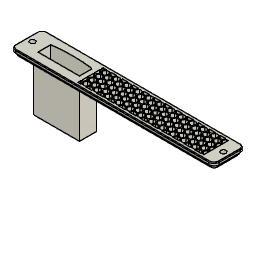
Front Vent -  SD_Card (Autodesk Fusion 360 design; units mm, degrees)
Autodesk Fusion 360 part; units mm, degrees
sketch "Sketch1" plane through (0, 0, 0) normal (0, 0, 1) x (1, 0, 0)
  line L0 (-84.9, 11.9) -> (84.9, 11.9)
  line L1 (84.9, 11.9) -> (84.9, -11.9)
  line L2 (84.9, -11.9) -> (-84.9, -11.9)
  line L3 (-84.9, -11.9) -> (-84.9, 11.9)
  circle A0 centre (-81.9, 8.9) radius 3
  circle A1 centre (-81.9, -8.9) radius 3
  circle A2 centre (81.9, 8.9) radius 3
  circle A3 centre (81.9, -8.9) radius 3
  line L4 (-107.1873, 0) -> (-105, 0)
  line L5 (-105, 0) -> (105, 0) construction
  circle A4 centre (-81, 0) radius 2.2
  circle A5 centre (81, 0) radius 2.2
  dimension "d21_3_1" = 169.8
  dimension "d22_3_1" = 84.9
  dimension "d23_3_1" = 23.8
  dimension "d24_3_1" = 11.9
  dimension "d25_3_1" = 6
  dimension "d26_3_1" = 6
  dimension "d27_3_1" = 6
  dimension "d28_3_1" = 6
  dimension "d29_3_1" = 210
  dimension "d30_3_1" = 4.4
  dimension "d31_3_1" = 4.4
  dimension "d32_3_1" = 3.9
  dimension "d33_3_1" = 3.9
  constraint horizontal L0
  constraint vertical L1
  constraint horizontal L2
  constraint vertical L3
  constraint tangent L0 A0
  constraint tangent L3 A0
  constraint tangent L2 A1
  constraint tangent L3 A1
  constraint tangent L2 A3
  constraint tangent L0 A2
  constraint tangent L1 A2
  constraint tangent L1 A3
  constraint parallel L2 L4
  constraint parallel L2 L5
  constraint midpoint origin L5
  constraint coincident L5 A4.centre
  constraint coincident L5 A5.centre
  measures "d21_3_1" distance of L0.start L0.end
  measures "d22_3_1" distance of origin L3
  measures "d23_3_1" distance of L0.start L2.end
  measures "d24_3_1" distance of origin L0
  measures "d25_3_1" diameter of A0
  measures "d26_3_1" diameter of A1
  measures "d27_3_1" diameter of A2
  measures "d28_3_1" diameter of A3
  measures "d29_3_1" distance of L4.end L5.end
  measures "d30_3_1" diameter of A4
  measures "d31_3_1" diameter of A5
  measures "d32_3_1" distance of L3 A4.centre
  measures "d33_3_1" distance of L1 A5.centre
extrude "Extrude1" add sketch "Sketch1" along normal blind 2.8 contours L0 L1 L2 L3 A0 A1 A2 A3 | A0 | A2 | A1 | A3
sketch "Sketch2" plane through (0, 0, 2.8) normal (0, 0, 1) x (-1, 0, 0)
  circle A0 centre (81, 0) radius 2.2
  circle A1 centre (-81, 0) radius 2.2
  arc A2 (81.9, -11.9) -> (84.9, -8.9) centre (81.9, -8.9) ccw
  line L0 (84.9, -8.9) -> (84.9, 8.9)
  arc A3 (84.9, 8.9) -> (81.9, 11.9) centre (81.9, 8.9) ccw
  line L1 (81.9, 11.9) -> (-81.9, 11.9)
  arc A4 (-81.9, 11.9) -> (-84.9, 8.9) centre (-81.9, 8.9) ccw
  line L2 (-84.9, 8.9) -> (-84.9, -8.9)
  arc A5 (-84.9, -8.9) -> (-81.9, -11.9) centre (-81.9, -8.9) ccw
  line L3 (-81.9, -11.9) -> (81.9, -11.9)
  line L4 (-81.9, -13.3) -> (81.9, -13.3)
  arc A6 (81.9, -13.3) -> (86.3, -8.9) centre (81.9, -8.9) ccw
  line L5 (86.3, -8.9) -> (86.3, 8.9)
  arc A7 (86.3, 8.9) -> (81.9, 13.3) centre (81.9, 8.9) ccw
  line L6 (81.9, 13.3) -> (-81.9, 13.3)
  arc A8 (-81.9, 13.3) -> (-86.3, 8.9) centre (-81.9, 8.9) ccw
  line L7 (-86.3, 8.9) -> (-86.3, -8.9)
  arc A9 (-86.3, -8.9) -> (-81.9, -13.3) centre (-81.9, -8.9) ccw
  dimension "d36_3_1" = 1.4
extrude "Extrude2" add sketch "Sketch2" along normal blind 2.4 contours A2 L0 A3 L1 A4 L2 A5 L3 | L4 A6 L5 A7 L6 A8 L7 A9
chamfer "Chamfer1" distance 0.6 angle 45 8 edges at (86.3, 0, 5.2) (85.0113, 12.0113, 5.2) (0, 13.3, 5.2) (-85.0113, 12.0113, 5.2) (-86.3, 0, 5.2) (-85.0113, -12.0113, 5.2) (0, -13.3, 5.2) (85.0113, -12.0113, 5.2)
sketch "Sketch4" plane through (-1.7827, -2.3697, 0) normal (0, 0, -1) x (1, 0, 0)
  circle A0 centre (-79.2173, -2.3697) radius 2.2
  circle A1 centre (82.7827, -2.3697) radius 2.2
  arc A2 (-83.1173, -11.2697) -> (-80.1173, -14.2697) centre (-80.1173, -11.2697) ccw
  line L0 (-80.1173, -14.2697) -> (83.6827, -14.2697)
  arc A3 (83.6827, -14.2697) -> (86.6827, -11.2697) centre (83.6827, -11.2697) ccw
  line L1 (86.6827, -11.2697) -> (86.6827, 6.5303)
  arc A4 (86.6827, 6.5303) -> (83.6827, 9.5303) centre (83.6827, 6.5303) ccw
  line L2 (83.6827, 9.5303) -> (-80.1173, 9.5303)
  arc A5 (-80.1173, 9.5303) -> (-83.1173, 6.5303) centre (-80.1173, 6.5303) ccw
  line L3 (-83.1173, 6.5303) -> (-83.1173, -11.2697)
  line L4 (-82.6173, 6.5303) -> (-82.6173, -11.2697)
  arc A6 (-82.6173, -11.2697) -> (-80.1173, -13.7697) centre (-80.1173, -11.2697) ccw
  line L5 (-80.1173, -13.7697) -> (83.6827, -13.7697)
  arc A7 (83.6827, -13.7697) -> (86.1827, -11.2697) centre (83.6827, -11.2697) ccw
  line L6 (86.1827, -11.2697) -> (86.1827, 6.5303)
  arc A8 (86.1827, 6.5303) -> (83.6827, 9.0303) centre (83.6827, 6.5303) ccw
  line L7 (83.6827, 9.0303) -> (-80.1173, 9.0303)
  arc A9 (-80.1173, 9.0303) -> (-82.6173, 6.5303) centre (-80.1173, 6.5303) ccw
  dimension "d44_3_1" = -0.5
extrude "Extrude4" cut sketch "Sketch4" against normal up to surface (2.8 mm away) contours A2 L0 A3 L1 A4 L2 A5 L3
sketch "Sketch6" plane through (0, 0, 5.2) normal (0, 0, 1) x (-1, 0, 0)
  circle A0 centre (81, 0) radius 2.2
  circle A1 centre (-81, 0) radius 2.2
  line L0 (-85.7, 8.9) -> (-85.7, -8.9)
  arc A2 (-85.7, -8.9) -> (-81.9, -12.7) centre (-81.9, -8.9) ccw
  line L1 (-81.9, -12.7) -> (81.9, -12.7)
  arc A3 (81.9, -12.7) -> (85.7, -8.9) centre (81.9, -8.9) ccw
  line L2 (85.7, -8.9) -> (85.7, 8.9)
  arc A4 (85.7, 8.9) -> (81.9, 12.7) centre (81.9, 8.9) ccw
  line L3 (81.9, 12.7) -> (-81.9, 12.7)
  arc A5 (-81.9, 12.7) -> (-85.7, 8.9) centre (-81.9, 8.9) ccw
  line L4 (71, -5.4) -> (35.8, -5.4)
  line L5 (35.8, -5.4) -> (35.8, 5.4)
  line L6 (35.8, 5.4) -> (71, 5.4)
  line L7 (71, 5.4) -> (71, -5.4)
  arc A6 (35.8, -5.4) -> (71, -5.4) centre (53.4, 123.0667) ccw
  arc A7 (33.8, -7.133) -> (73, -7.133) centre (53.4, 123.0667) ccw
  line L8 (73, 7.4) -> (73, -7.133)
  line L9 (33.8, 7.4) -> (73, 7.4)
  line L10 (33.8, -7.133) -> (33.8, 7.4)
  point P0 (81, 0)
  point P1 (71, 0)
  point P2 (53.4, 5.4)
  point P3 (53.4, -6.6)
  dimension "d323_1" = 12
  dimension "d324_1" = 10.8
  dimension "d325_1" = 10
  dimension "d326_1" = 2
  dimension "d337_1" = 35.2
  constraint horizontal L4
  constraint vertical L5
  constraint horizontal L6
  constraint vertical L7
  constraint coincident P0 A0.centre
  constraint midpoint L7 P1
  constraint midpoint L6 P2
  constraint midpoint A6 P3
  constraint horizontal P0 P1
  measures "d323_1" distance of P2 P3
  measures "d324_1" distance of L4.end L5.end
  measures "d325_1" distance of P0 P1
  measures "d337_1" distance of L5 L7
extrude "Extrude16" cut sketch "Sketch6" against normal blind 10 contours L4 A6
extrude "Extrude10" cut sketch "Sketch6" against normal blind 5.2 contours L4 L5 L6 L7
extrude "Extrude9" add sketch "Sketch6" against normal blind 44 contours A7 L8 L9 L10
sketch "Sketch7" plane through (0, 0, -38.8) normal (0, 0, -1) x (1, 0, 0)
  line L0 (-35.8, 5.4) -> (-35.8, -5.4)
  arc A0 (-71, -5.4) -> (-35.8, -5.4) centre (-53.4, 123.0667) ccw
  line L1 (-71, -5.4) -> (-71, 5.4)
  line L2 (-71, 5.4) -> (-35.8, 5.4)
  arc A1 (-73, -7.133) -> (-33.8, -7.133) centre (-53.4, 123.0667) ccw
  line L3 (-33.8, -7.133) -> (-33.8, 7.4)
  line L4 (-33.8, 7.4) -> (-73, 7.4)
  line L5 (-73, 7.4) -> (-73, -7.133)
extrude "Extrude11" add sketch "Sketch7" along normal blind 2 contours L0 A0 L1 L2 | A1 L3 L4 L5
sketch "Sketch8" plane through (0, 0, -40.8) normal (0, 0, -1) x (1, 0, 0)
  line L0 (-73, 7.4) -> (-73, -7.133)
  arc A0 (-73, -7.133) -> (-33.8, -7.133) centre (-53.4, 123.0667) ccw
  line L1 (-33.8, -7.133) -> (-33.8, 7.4)
  line L2 (-64.4, 2) -> (-42.4, 2)
  line L3 (-42.4, 2) -> (-42.4, -2)
  line L4 (-42.4, -2) -> (-64.4, -2)
  line L5 (-64.4, -2) -> (-64.4, 2)
  point P0 (-81, 0)
  point P1 (-64.4, 0)
  point P2 (-53.4, 2)
  point P3 (-53.4, 5.4)
  dimension "d335_1" = 13.8426
  dimension "d336_1" = 22
  dimension "d338_1" = 4
  constraint horizontal L2
  constraint vertical L3
  constraint horizontal L4
  constraint vertical L5
  constraint midpoint L5 P1
  constraint horizontal P0 P1
  constraint midpoint L2 P2
  constraint vertical P2 P3
  measures "d336_1" distance of L2.start L2.end
  measures "d338_1" distance of L2.end L3.end
extrude "Extrude12" cut sketch "Sketch8" against normal blind 2
fillet "Fillet1" radius 1 4 edges at (-64.4, -2, -39.8) (-42.4, -2, -39.8) (-42.4, 2, -39.8) (-64.4, 2, -39.8)
sketch "Sketch10" plane through (0, 0, 5.2) normal (0, 0, 1) x (-1, 0, 0)
  line L0 (31.8, -10.7) -> (-75, -10.7)
  line L1 (-75, -10.7) -> (-75, 10.7)
  line L2 (-75, 10.7) -> (31.8, 10.7)
  line L3 (31.8, 10.7) -> (31.8, -10.7)
  line L4 (33.8, -7.133) -> (33.8, 7.4)
  line L5 (-21.6, -10.7) -> (-21.6, 10.7) construction
  line L6 (81.9, 12.7) -> (-81.9, 12.7)
  line L7 (-81.9, -12.7) -> (81.9, -12.7)
  line L8 (29.1731, 0) -> (30.4865, -2.275)
  line L9 (30.4865, -2.275) -> (33.1135, -2.275)
  line L10 (33.1135, -2.275) -> (34.4269, 0)
  line L11 (34.4269, 0) -> (33.1135, 2.275)
  line L12 (33.1135, 2.275) -> (30.4865, 2.275)
  line L13 (30.4865, 2.275) -> (29.1731, 0)
  line L14 (31.8, 0) -> (29.0768, 0)
  line L15 (29.0768, 0) -> (-75, 0) construction
  line L16 (30.4865, -3.075) -> (29.1731, -5.35)
  line L17 (29.1731, -5.35) -> (30.4865, -7.625)
  line L18 (30.4865, -7.625) -> (33.1135, -7.625)
  line L19 (33.1135, -7.625) -> (34.4269, -5.35)
  line L20 (34.4269, -5.35) -> (33.1135, -3.075)
  line L21 (33.1135, -3.075) -> (30.4865, -3.075)
  line L22 (29.1731, -10.7) -> (30.4865, -12.975)
  line L23 (30.4865, -12.975) -> (33.1135, -12.975)
  line L24 (33.1135, -12.975) -> (34.4269, -10.7)
  line L25 (34.4269, -10.7) -> (33.1135, -8.425)
  line L26 (33.1135, -8.425) -> (30.4865, -8.425)
  line L27 (30.4865, -8.425) -> (29.1731, -10.7)
  line L28 (29.1731, 5.35) -> (30.4865, 3.075)
  line L29 (30.4865, 3.075) -> (33.1135, 3.075)
  line L30 (33.1135, 3.075) -> (34.4269, 5.35)
  line L31 (34.4269, 5.35) -> (33.1135, 7.625)
  line L32 (33.1135, 7.625) -> (30.4865, 7.625)
  line L33 (30.4865, 7.625) -> (29.1731, 5.35)
  line L34 (30.4865, 12.975) -> (29.1731, 10.7)
  line L35 (29.1731, 10.7) -> (30.4865, 8.425)
  line L36 (30.4865, 8.425) -> (33.1135, 8.425)
  line L37 (33.1135, 8.425) -> (34.4269, 10.7)
  line L38 (34.4269, 10.7) -> (33.1135, 12.975)
  line L39 (33.1135, 12.975) -> (30.4865, 12.975)
  line L40 (24.5398, -8.025) -> (25.8533, -10.3)
  line L41 (25.8533, -10.3) -> (28.4802, -10.3)
  line L42 (28.4802, -10.3) -> (29.7937, -8.025)
  line L43 (29.7937, -8.025) -> (28.4802, -5.75)
  line L44 (28.4802, -5.75) -> (25.8533, -5.75)
  line L45 (25.8533, -5.75) -> (24.5398, -8.025)
  line L46 (24.5398, -2.675) -> (25.8533, -4.95)
  line L47 (25.8533, -4.95) -> (28.4802, -4.95)
  line L48 (28.4802, -4.95) -> (29.7937, -2.675)
  line L49 (29.7937, -2.675) -> (28.4802, -0.4)
  line L50 (28.4802, -0.4) -> (25.8533, -0.4)
  line L51 (25.8533, -0.4) -> (24.5398, -2.675)
  line L52 (24.5398, 2.675) -> (25.8533, 0.4)
  line L53 (25.8533, 0.4) -> (28.4802, 0.4)
  line L54 (28.4802, 0.4) -> (29.7937, 2.675)
  line L55 (29.7937, 2.675) -> (28.4802, 4.95)
  line L56 (28.4802, 4.95) -> (25.8533, 4.95)
  line L57 (25.8533, 4.95) -> (24.5398, 2.675)
  line L58 (24.5398, 8.025) -> (25.8533, 5.75)
  line L59 (25.8533, 5.75) -> (28.4802, 5.75)
  line L60 (28.4802, 5.75) -> (29.7937, 8.025)
  line L61 (29.7937, 8.025) -> (28.4802, 10.3)
  line L62 (28.4802, 10.3) -> (25.8533, 10.3)
  line L63 (25.8533, 10.3) -> (24.5398, 8.025)
  line L64 (27.1668, -10.7) -> (27.1668, 10.7) construction
  line L65 (7.8533, -10.3) -> (10.4802, -10.3)
  line L66 (-1.1467, -10.3) -> (1.4802, -10.3)
  line L67 (21.2205, 8.425) -> (23.8475, 8.425)
  line L68 (23.8475, 8.425) -> (25.1609, 10.7)
  line L69 (25.1609, 10.7) -> (23.8475, 12.975)
  line L70 (23.8475, 12.975) -> (21.2205, 12.975)
  line L71 (19.9071, 10.7) -> (21.2205, 8.425)
  line L72 (21.2205, 12.975) -> (19.9071, 10.7)
  line L73 (16.5873, 5.75) -> (19.2142, 5.75)
  line L74 (19.2142, 5.75) -> (20.5277, 8.025)
  line L75 (20.5277, 8.025) -> (19.2142, 10.3)
  line L76 (19.2142, 10.3) -> (16.5873, 10.3)
  line L77 (15.2738, 8.025) -> (16.5873, 5.75)
  line L78 (16.5873, 10.3) -> (15.2738, 8.025)
  line L79 (19.9071, 5.35) -> (21.2205, 3.075)
  line L80 (21.2205, 3.075) -> (23.8475, 3.075)
  line L81 (23.8475, 3.075) -> (25.1609, 5.35)
  line L82 (25.1609, 5.35) -> (23.8475, 7.625)
  line L83 (21.2205, 7.625) -> (19.9071, 5.35)
  line L84 (23.8475, 7.625) -> (21.2205, 7.625)
  line L85 (16.5873, 0.4) -> (19.2142, 0.4)
  line L86 (19.2142, 0.4) -> (20.5277, 2.675)
  line L87 (20.5277, 2.675) -> (19.2142, 4.95)
  line L88 (19.2142, 4.95) -> (16.5873, 4.95)
  line L89 (15.2738, 2.675) -> (16.5873, 0.4)
  line L90 (16.5873, 4.95) -> (15.2738, 2.675)
  line L91 (21.2205, -2.275) -> (23.8475, -2.275)
  line L92 (23.8475, -2.275) -> (25.1609, 0)
  line L93 (25.1609, 0) -> (23.8475, 2.275)
  line L94 (23.8475, 2.275) -> (21.2205, 2.275)
  line L95 (19.9071, 0) -> (21.2205, -2.275)
  line L96 (21.2205, 2.275) -> (19.9071, 0)
  line L97 (16.5873, -0.4) -> (15.2738, -2.675)
  line L98 (15.2738, -2.675) -> (16.5873, -4.95)
  line L99 (16.5873, -4.95) -> (19.2142, -4.95)
  line L100 (19.2142, -4.95) -> (20.5277, -2.675)
  line L101 (19.2142, -0.4) -> (16.5873, -0.4)
  line L102 (20.5277, -2.675) -> (19.2142, -0.4)
  line L103 (21.2205, -7.625) -> (23.8475, -7.625)
  line L104 (23.8475, -7.625) -> (25.1609, -5.35)
  line L105 (25.1609, -5.35) -> (23.8475, -3.075)
  line L106 (23.8475, -3.075) -> (21.2205, -3.075)
  line L107 (19.9071, -5.35) -> (21.2205, -7.625)
  line L108 (21.2205, -3.075) -> (19.9071, -5.35)
  line L109 (16.5873, -5.75) -> (15.2738, -8.025)
  line L110 (15.2738, -8.025) -> (16.5873, -10.3)
  line L111 (16.5873, -10.3) -> (19.2142, -10.3)
  line L112 (19.2142, -10.3) -> (20.5277, -8.025)
  line L113 (19.2142, -5.75) -> (16.5873, -5.75)
  line L114 (20.5277, -8.025) -> (19.2142, -5.75)
  line L115 (21.2205, -12.975) -> (23.8475, -12.975)
  line L116 (23.8475, -12.975) -> (25.1609, -10.7)
  line L117 (25.1609, -10.7) -> (23.8475, -8.425)
  line L118 (23.8475, -8.425) -> (21.2205, -8.425)
  line L119 (19.9071, -10.7) -> (21.2205, -12.975)
  line L120 (21.2205, -8.425) -> (19.9071, -10.7)
  line L121 (11.9545, 8.425) -> (14.5815, 8.425)
  line L122 (14.5815, 8.425) -> (15.8949, 10.7)
  line L123 (15.8949, 10.7) -> (14.5815, 12.975)
  line L124 (14.5815, 12.975) -> (11.9545, 12.975)
  line L125 (10.6411, 10.7) -> (11.9545, 8.425)
  line L126 (11.9545, 12.975) -> (10.6411, 10.7)
  line L127 (7.3213, 5.75) -> (9.9482, 5.75)
  line L128 (9.9482, 5.75) -> (11.2617, 8.025)
  line L129 (11.2617, 8.025) -> (9.9482, 10.3)
  line L130 (9.9482, 10.3) -> (7.3213, 10.3)
  line L131 (6.0078, 8.025) -> (7.3213, 5.75)
  line L132 (7.3213, 10.3) -> (6.0078, 8.025)
  line L133 (10.6411, 5.35) -> (11.9545, 3.075)
  line L134 (11.9545, 3.075) -> (14.5815, 3.075)
  line L135 (14.5815, 3.075) -> (15.8949, 5.35)
  line L136 (15.8949, 5.35) -> (14.5815, 7.625)
  line L137 (11.9545, 7.625) -> (10.6411, 5.35)
  line L138 (14.5815, 7.625) -> (11.9545, 7.625)
  line L139 (7.3213, 0.4) -> (9.9482, 0.4)
  line L140 (9.9482, 0.4) -> (11.2617, 2.675)
  line L141 (11.2617, 2.675) -> (9.9482, 4.95)
  line L142 (9.9482, 4.95) -> (7.3213, 4.95)
  line L143 (6.0078, 2.675) -> (7.3213, 0.4)
  line L144 (7.3213, 4.95) -> (6.0078, 2.675)
  line L145 (11.9545, -2.275) -> (14.5815, -2.275)
  line L146 (14.5815, -2.275) -> (15.8949, 0)
  line L147 (15.8949, 0) -> (14.5815, 2.275)
  line L148 (14.5815, 2.275) -> (11.9545, 2.275)
  line L149 (10.6411, 0) -> (11.9545, -2.275)
  line L150 (11.9545, 2.275) -> (10.6411, 0)
  line L151 (7.3213, -0.4) -> (6.0078, -2.675)
  line L152 (6.0078, -2.675) -> (7.3213, -4.95)
  line L153 (7.3213, -4.95) -> (9.9482, -4.95)
  line L154 (9.9482, -4.95) -> (11.2617, -2.675)
  line L155 (9.9482, -0.4) -> (7.3213, -0.4)
  line L156 (11.2617, -2.675) -> (9.9482, -0.4)
  line L157 (11.9545, -7.625) -> (14.5815, -7.625)
  line L158 (14.5815, -7.625) -> (15.8949, -5.35)
  line L159 (15.8949, -5.35) -> (14.5815, -3.075)
  line L160 (14.5815, -3.075) -> (11.9545, -3.075)
  line L161 (10.6411, -5.35) -> (11.9545, -7.625)
  line L162 (11.9545, -3.075) -> (10.6411, -5.35)
  line L163 (7.3213, -5.75) -> (6.0078, -8.025)
  line L164 (6.0078, -8.025) -> (7.3213, -10.3)
  line L165 (7.3213, -10.3) -> (9.9482, -10.3)
  line L166 (9.9482, -10.3) -> (11.2617, -8.025)
  line L167 (9.9482, -5.75) -> (7.3213, -5.75)
  line L168 (11.2617, -8.025) -> (9.9482, -5.75)
  line L169 (11.9545, -12.975) -> (14.5815, -12.975)
  line L170 (14.5815, -12.975) -> (15.8949, -10.7)
  line L171 (15.8949, -10.7) -> (14.5815, -8.425)
  line L172 (14.5815, -8.425) -> (11.9545, -8.425)
  line L173 (10.6411, -10.7) -> (11.9545, -12.975)
  line L174 (11.9545, -8.425) -> (10.6411, -10.7)
  line L175 (2.6885, 8.425) -> (5.3155, 8.425)
  line L176 (5.3155, 8.425) -> (6.6289, 10.7)
  line L177 (6.6289, 10.7) -> (5.3155, 12.975)
  line L178 (5.3155, 12.975) -> (2.6885, 12.975)
  line L179 (1.3751, 10.7) -> (2.6885, 8.425)
  line L180 (2.6885, 12.975) -> (1.3751, 10.7)
  line L181 (-1.9447, 5.75) -> (0.6822, 5.75)
  line L182 (0.6822, 5.75) -> (1.9957, 8.025)
  line L183 (1.9957, 8.025) -> (0.6822, 10.3)
  line L184 (0.6822, 10.3) -> (-1.9447, 10.3)
  line L185 (-3.2582, 8.025) -> (-1.9447, 5.75)
  line L186 (-1.9447, 10.3) -> (-3.2582, 8.025)
  line L187 (1.3751, 5.35) -> (2.6885, 3.075)
  line L188 (2.6885, 3.075) -> (5.3155, 3.075)
  line L189 (5.3155, 3.075) -> (6.6289, 5.35)
  line L190 (6.6289, 5.35) -> (5.3155, 7.625)
  line L191 (2.6885, 7.625) -> (1.3751, 5.35)
  line L192 (5.3155, 7.625) -> (2.6885, 7.625)
  line L193 (-1.9447, 0.4) -> (0.6822, 0.4)
  line L194 (0.6822, 0.4) -> (1.9957, 2.675)
  line L195 (1.9957, 2.675) -> (0.6822, 4.95)
  line L196 (0.6822, 4.95) -> (-1.9447, 4.95)
  line L197 (-3.2582, 2.675) -> (-1.9447, 0.4)
  line L198 (-1.9447, 4.95) -> (-3.2582, 2.675)
  line L199 (2.6885, -2.275) -> (5.3155, -2.275)
  line L200 (5.3155, -2.275) -> (6.6289, 0)
  line L201 (6.6289, 0) -> (5.3155, 2.275)
  line L202 (5.3155, 2.275) -> (2.6885, 2.275)
  line L203 (1.3751, 0) -> (2.6885, -2.275)
  line L204 (2.6885, 2.275) -> (1.3751, 0)
  line L205 (-1.9447, -0.4) -> (-3.2582, -2.675)
  line L206 (-3.2582, -2.675) -> (-1.9447, -4.95)
  line L207 (-1.9447, -4.95) -> (0.6822, -4.95)
  line L208 (0.6822, -4.95) -> (1.9957, -2.675)
  line L209 (0.6822, -0.4) -> (-1.9447, -0.4)
  line L210 (1.9957, -2.675) -> (0.6822, -0.4)
  line L211 (2.6885, -7.625) -> (5.3155, -7.625)
  line L212 (5.3155, -7.625) -> (6.6289, -5.35)
  line L213 (6.6289, -5.35) -> (5.3155, -3.075)
  line L214 (5.3155, -3.075) -> (2.6885, -3.075)
  line L215 (1.3751, -5.35) -> (2.6885, -7.625)
  line L216 (2.6885, -3.075) -> (1.3751, -5.35)
  line L217 (-1.9447, -5.75) -> (-3.2582, -8.025)
  line L218 (-3.2582, -8.025) -> (-1.9447, -10.3)
  line L219 (-1.9447, -10.3) -> (0.6822, -10.3)
  line L220 (0.6822, -10.3) -> (1.9957, -8.025)
  line L221 (0.6822, -5.75) -> (-1.9447, -5.75)
  line L222 (1.9957, -8.025) -> (0.6822, -5.75)
  line L223 (2.6885, -12.975) -> (5.3155, -12.975)
  line L224 (5.3155, -12.975) -> (6.6289, -10.7)
  line L225 (6.6289, -10.7) -> (5.3155, -8.425)
  line L226 (5.3155, -8.425) -> (2.6885, -8.425)
  line L227 (1.3751, -10.7) -> (2.6885, -12.975)
  line L228 (2.6885, -8.425) -> (1.3751, -10.7)
  line L229 (-6.5775, 8.425) -> (-3.9505, 8.425)
  line L230 (-3.9505, 8.425) -> (-2.6371, 10.7)
  line L231 (-2.6371, 10.7) -> (-3.9505, 12.975)
  line L232 (-3.9505, 12.975) -> (-6.5775, 12.975)
  line L233 (-7.8909, 10.7) -> (-6.5775, 8.425)
  line L234 (-6.5775, 12.975) -> (-7.8909, 10.7)
  line L235 (-11.2107, 5.75) -> (-8.5838, 5.75)
  line L236 (-8.5838, 5.75) -> (-7.2703, 8.025)
  line L237 (-7.2703, 8.025) -> (-8.5838, 10.3)
  line L238 (-8.5838, 10.3) -> (-11.2107, 10.3)
  line L239 (-12.5242, 8.025) -> (-11.2107, 5.75)
  line L240 (-11.2107, 10.3) -> (-12.5242, 8.025)
  line L241 (-7.8909, 5.35) -> (-6.5775, 3.075)
  line L242 (-6.5775, 3.075) -> (-3.9505, 3.075)
  line L243 (-3.9505, 3.075) -> (-2.6371, 5.35)
  line L244 (-2.6371, 5.35) -> (-3.9505, 7.625)
  line L245 (-6.5775, 7.625) -> (-7.8909, 5.35)
  line L246 (-3.9505, 7.625) -> (-6.5775, 7.625)
  line L247 (-11.2107, 0.4) -> (-8.5838, 0.4)
  line L248 (-8.5838, 0.4) -> (-7.2703, 2.675)
  line L249 (-7.2703, 2.675) -> (-8.5838, 4.95)
  line L250 (-8.5838, 4.95) -> (-11.2107, 4.95)
  line L251 (-12.5242, 2.675) -> (-11.2107, 0.4)
  line L252 (-11.2107, 4.95) -> (-12.5242, 2.675)
  line L253 (-6.5775, -2.275) -> (-3.9505, -2.275)
  line L254 (-3.9505, -2.275) -> (-2.6371, 0)
  line L255 (-2.6371, 0) -> (-3.9505, 2.275)
  line L256 (-3.9505, 2.275) -> (-6.5775, 2.275)
  line L257 (-7.8909, 0) -> (-6.5775, -2.275)
  line L258 (-6.5775, 2.275) -> (-7.8909, 0)
  line L259 (-11.2107, -0.4) -> (-12.5242, -2.675)
  line L260 (-12.5242, -2.675) -> (-11.2107, -4.95)
  line L261 (-11.2107, -4.95) -> (-8.5838, -4.95)
  line L262 (-8.5838, -4.95) -> (-7.2703, -2.675)
  line L263 (-8.5838, -0.4) -> (-11.2107, -0.4)
  line L264 (-7.2703, -2.675) -> (-8.5838, -0.4)
  line L265 (-6.5775, -7.625) -> (-3.9505, -7.625)
  line L266 (-3.9505, -7.625) -> (-2.6371, -5.35)
  line L267 (-2.6371, -5.35) -> (-3.9505, -3.075)
  line L268 (-3.9505, -3.075) -> (-6.5775, -3.075)
  line L269 (-7.8909, -5.35) -> (-6.5775, -7.625)
  line L270 (-6.5775, -3.075) -> (-7.8909, -5.35)
  line L271 (-11.2107, -5.75) -> (-12.5242, -8.025)
  line L272 (-12.5242, -8.025) -> (-11.2107, -10.3)
  line L273 (-11.2107, -10.3) -> (-8.5838, -10.3)
  line L274 (-8.5838, -10.3) -> (-7.2703, -8.025)
  line L275 (-8.5838, -5.75) -> (-11.2107, -5.75)
  line L276 (-7.2703, -8.025) -> (-8.5838, -5.75)
  line L277 (-6.5775, -12.975) -> (-3.9505, -12.975)
  line L278 (-3.9505, -12.975) -> (-2.6371, -10.7)
  line L279 (-2.6371, -10.7) -> (-3.9505, -8.425)
  line L280 (-3.9505, -8.425) -> (-6.5775, -8.425)
  line L281 (-7.8909, -10.7) -> (-6.5775, -12.975)
  line L282 (-6.5775, -8.425) -> (-7.8909, -10.7)
  line L283 (-15.8435, 8.425) -> (-13.2165, 8.425)
  line L284 (-13.2165, 8.425) -> (-11.9031, 10.7)
  line L285 (-11.9031, 10.7) -> (-13.2165, 12.975)
  line L286 (-13.2165, 12.975) -> (-15.8435, 12.975)
  line L287 (-17.1569, 10.7) -> (-15.8435, 8.425)
  line L288 (-15.8435, 12.975) -> (-17.1569, 10.7)
  line L289 (-20.4767, 5.75) -> (-17.8498, 5.75)
  line L290 (-17.8498, 5.75) -> (-16.5363, 8.025)
  line L291 (-16.5363, 8.025) -> (-17.8498, 10.3)
  line L292 (-17.8498, 10.3) -> (-20.4767, 10.3)
  line L293 (-21.7902, 8.025) -> (-20.4767, 5.75)
  line L294 (-20.4767, 10.3) -> (-21.7902, 8.025)
  line L295 (-17.1569, 5.35) -> (-15.8435, 3.075)
  line L296 (-15.8435, 3.075) -> (-13.2165, 3.075)
  line L297 (-13.2165, 3.075) -> (-11.9031, 5.35)
  line L298 (-11.9031, 5.35) -> (-13.2165, 7.625)
  line L299 (-15.8435, 7.625) -> (-17.1569, 5.35)
  line L300 (-13.2165, 7.625) -> (-15.8435, 7.625)
  line L301 (-20.4767, 0.4) -> (-17.8498, 0.4)
  line L302 (-17.8498, 0.4) -> (-16.5363, 2.675)
  line L303 (-16.5363, 2.675) -> (-17.8498, 4.95)
  line L304 (-17.8498, 4.95) -> (-20.4767, 4.95)
  line L305 (-21.7902, 2.675) -> (-20.4767, 0.4)
  line L306 (-20.4767, 4.95) -> (-21.7902, 2.675)
  line L307 (-15.8435, -2.275) -> (-13.2165, -2.275)
  line L308 (-13.2165, -2.275) -> (-11.9031, 0)
  line L309 (-11.9031, 0) -> (-13.2165, 2.275)
  line L310 (-13.2165, 2.275) -> (-15.8435, 2.275)
  line L311 (-17.1569, 0) -> (-15.8435, -2.275)
  line L312 (-15.8435, 2.275) -> (-17.1569, 0)
  line L313 (-20.4767, -0.4) -> (-21.7902, -2.675)
  line L314 (-21.7902, -2.675) -> (-20.4767, -4.95)
  line L315 (-20.4767, -4.95) -> (-17.8498, -4.95)
  line L316 (-17.8498, -4.95) -> (-16.5363, -2.675)
  line L317 (-17.8498, -0.4) -> (-20.4767, -0.4)
  line L318 (-16.5363, -2.675) -> (-17.8498, -0.4)
  line L319 (-15.8435, -7.625) -> (-13.2165, -7.625)
  line L320 (-13.2165, -7.625) -> (-11.9031, -5.35)
  line L321 (-11.9031, -5.35) -> (-13.2165, -3.075)
  line L322 (-13.2165, -3.075) -> (-15.8435, -3.075)
  line L323 (-17.1569, -5.35) -> (-15.8435, -7.625)
  line L324 (-15.8435, -3.075) -> (-17.1569, -5.35)
  line L325 (-20.4767, -5.75) -> (-21.7902, -8.025)
  line L326 (-21.7902, -8.025) -> (-20.4767, -10.3)
  line L327 (-20.4767, -10.3) -> (-17.8498, -10.3)
  line L328 (-17.8498, -10.3) -> (-16.5363, -8.025)
  line L329 (-17.8498, -5.75) -> (-20.4767, -5.75)
  line L330 (-16.5363, -8.025) -> (-17.8498, -5.75)
  line L331 (-15.8435, -12.975) -> (-13.2165, -12.975)
  line L332 (-13.2165, -12.975) -> (-11.9031, -10.7)
  line L333 (-11.9031, -10.7) -> (-13.2165, -8.425)
  line L334 (-13.2165, -8.425) -> (-15.8435, -8.425)
  line L335 (-17.1569, -10.7) -> (-15.8435, -12.975)
  line L336 (-15.8435, -8.425) -> (-17.1569, -10.7)
  line L337 (-25.1095, 8.425) -> (-22.4825, 8.425)
  line L338 (-22.4825, 8.425) -> (-21.1691, 10.7)
  line L339 (-21.1691, 10.7) -> (-22.4825, 12.975)
  line L340 (-22.4825, 12.975) -> (-25.1095, 12.975)
  line L341 (-26.4229, 10.7) -> (-25.1095, 8.425)
  line L342 (-25.1095, 12.975) -> (-26.4229, 10.7)
  line L343 (-29.7427, 5.75) -> (-27.1158, 5.75)
  line L344 (-27.1158, 5.75) -> (-25.8023, 8.025)
  line L345 (-25.8023, 8.025) -> (-27.1158, 10.3)
  line L346 (-27.1158, 10.3) -> (-29.7427, 10.3)
  line L347 (-31.0562, 8.025) -> (-29.7427, 5.75)
  line L348 (-29.7427, 10.3) -> (-31.0562, 8.025)
  line L349 (-26.4229, 5.35) -> (-25.1095, 3.075)
  line L350 (-25.1095, 3.075) -> (-22.4825, 3.075)
  line L351 (-22.4825, 3.075) -> (-21.1691, 5.35)
  line L352 (-21.1691, 5.35) -> (-22.4825, 7.625)
  line L353 (-25.1095, 7.625) -> (-26.4229, 5.35)
  line L354 (-22.4825, 7.625) -> (-25.1095, 7.625)
  line L355 (-29.7427, 0.4) -> (-27.1158, 0.4)
  line L356 (-27.1158, 0.4) -> (-25.8023, 2.675)
  line L357 (-25.8023, 2.675) -> (-27.1158, 4.95)
  line L358 (-27.1158, 4.95) -> (-29.7427, 4.95)
  line L359 (-31.0562, 2.675) -> (-29.7427, 0.4)
  line L360 (-29.7427, 4.95) -> (-31.0562, 2.675)
  line L361 (-25.1095, -2.275) -> (-22.4825, -2.275)
  line L362 (-22.4825, -2.275) -> (-21.1691, 0)
  line L363 (-21.1691, 0) -> (-22.4825, 2.275)
  line L364 (-22.4825, 2.275) -> (-25.1095, 2.275)
  line L365 (-26.4229, 0) -> (-25.1095, -2.275)
  line L366 (-25.1095, 2.275) -> (-26.4229, 0)
  line L367 (-29.7427, -0.4) -> (-31.0562, -2.675)
  line L368 (-31.0562, -2.675) -> (-29.7427, -4.95)
  line L369 (-29.7427, -4.95) -> (-27.1158, -4.95)
  line L370 (-27.1158, -4.95) -> (-25.8023, -2.675)
  line L371 (-27.1158, -0.4) -> (-29.7427, -0.4)
  line L372 (-25.8023, -2.675) -> (-27.1158, -0.4)
  line L373 (-25.1095, -7.625) -> (-22.4825, -7.625)
  line L374 (-22.4825, -7.625) -> (-21.1691, -5.35)
  line L375 (-21.1691, -5.35) -> (-22.4825, -3.075)
  line L376 (-22.4825, -3.075) -> (-25.1095, -3.075)
  line L377 (-26.4229, -5.35) -> (-25.1095, -7.625)
  line L378 (-25.1095, -3.075) -> (-26.4229, -5.35)
  line L379 (-29.7427, -5.75) -> (-31.0562, -8.025)
  line L380 (-31.0562, -8.025) -> (-29.7427, -10.3)
  line L381 (-29.7427, -10.3) -> (-27.1158, -10.3)
  line L382 (-27.1158, -10.3) -> (-25.8023, -8.025)
  line L383 (-27.1158, -5.75) -> (-29.7427, -5.75)
  line L384 (-25.8023, -8.025) -> (-27.1158, -5.75)
  line L385 (-25.1095, -12.975) -> (-22.4825, -12.975)
  line L386 (-22.4825, -12.975) -> (-21.1691, -10.7)
  line L387 (-21.1691, -10.7) -> (-22.4825, -8.425)
  line L388 (-22.4825, -8.425) -> (-25.1095, -8.425)
  line L389 (-26.4229, -10.7) -> (-25.1095, -12.975)
  line L390 (-25.1095, -8.425) -> (-26.4229, -10.7)
  line L391 (-34.3755, 8.425) -> (-31.7485, 8.425)
  line L392 (-31.7485, 8.425) -> (-30.4351, 10.7)
  line L393 (-30.4351, 10.7) -> (-31.7485, 12.975)
  line L394 (-31.7485, 12.975) -> (-34.3755, 12.975)
  line L395 (-35.6889, 10.7) -> (-34.3755, 8.425)
  line L396 (-34.3755, 12.975) -> (-35.6889, 10.7)
  line L397 (-39.0087, 5.75) -> (-36.3818, 5.75)
  line L398 (-36.3818, 5.75) -> (-35.0683, 8.025)
  line L399 (-35.0683, 8.025) -> (-36.3818, 10.3)
  line L400 (-36.3818, 10.3) -> (-39.0087, 10.3)
  line L401 (-40.3222, 8.025) -> (-39.0087, 5.75)
  line L402 (-39.0087, 10.3) -> (-40.3222, 8.025)
  line L403 (-35.6889, 5.35) -> (-34.3755, 3.075)
  line L404 (-34.3755, 3.075) -> (-31.7485, 3.075)
  line L405 (-31.7485, 3.075) -> (-30.4351, 5.35)
  line L406 (-30.4351, 5.35) -> (-31.7485, 7.625)
  line L407 (-34.3755, 7.625) -> (-35.6889, 5.35)
  line L408 (-31.7485, 7.625) -> (-34.3755, 7.625)
  line L409 (-39.0087, 0.4) -> (-36.3818, 0.4)
  line L410 (-36.3818, 0.4) -> (-35.0683, 2.675)
  line L411 (-35.0683, 2.675) -> (-36.3818, 4.95)
  line L412 (-36.3818, 4.95) -> (-39.0087, 4.95)
  line L413 (-40.3222, 2.675) -> (-39.0087, 0.4)
  line L414 (-39.0087, 4.95) -> (-40.3222, 2.675)
  line L415 (-34.3755, -2.275) -> (-31.7485, -2.275)
  line L416 (-31.7485, -2.275) -> (-30.4351, 0)
  line L417 (-30.4351, 0) -> (-31.7485, 2.275)
  line L418 (-31.7485, 2.275) -> (-34.3755, 2.275)
  line L419 (-35.6889, 0) -> (-34.3755, -2.275)
  line L420 (-34.3755, 2.275) -> (-35.6889, 0)
  line L421 (-39.0087, -0.4) -> (-40.3222, -2.675)
  line L422 (-40.3222, -2.675) -> (-39.0087, -4.95)
  line L423 (-39.0087, -4.95) -> (-36.3818, -4.95)
  line L424 (-36.3818, -4.95) -> (-35.0683, -2.675)
  line L425 (-36.3818, -0.4) -> (-39.0087, -0.4)
  line L426 (-35.0683, -2.675) -> (-36.3818, -0.4)
  line L427 (-34.3755, -7.625) -> (-31.7485, -7.625)
  line L428 (-31.7485, -7.625) -> (-30.4351, -5.35)
  line L429 (-30.4351, -5.35) -> (-31.7485, -3.075)
  line L430 (-31.7485, -3.075) -> (-34.3755, -3.075)
  line L431 (-35.6889, -5.35) -> (-34.3755, -7.625)
  line L432 (-34.3755, -3.075) -> (-35.6889, -5.35)
  line L433 (-39.0087, -5.75) -> (-40.3222, -8.025)
  line L434 (-40.3222, -8.025) -> (-39.0087, -10.3)
  line L435 (-39.0087, -10.3) -> (-36.3818, -10.3)
  line L436 (-36.3818, -10.3) -> (-35.0683, -8.025)
  line L437 (-36.3818, -5.75) -> (-39.0087, -5.75)
  line L438 (-35.0683, -8.025) -> (-36.3818, -5.75)
  line L439 (-34.3755, -12.975) -> (-31.7485, -12.975)
  line L440 (-31.7485, -12.975) -> (-30.4351, -10.7)
  line L441 (-30.4351, -10.7) -> (-31.7485, -8.425)
  line L442 (-31.7485, -8.425) -> (-34.3755, -8.425)
  line L443 (-35.6889, -10.7) -> (-34.3755, -12.975)
  line L444 (-34.3755, -8.425) -> (-35.6889, -10.7)
  line L445 (-43.6415, 8.425) -> (-41.0145, 8.425)
  line L446 (-41.0145, 8.425) -> (-39.7011, 10.7)
  line L447 (-39.7011, 10.7) -> (-41.0145, 12.975)
  line L448 (-41.0145, 12.975) -> (-43.6415, 12.975)
  line L449 (-44.9549, 10.7) -> (-43.6415, 8.425)
  line L450 (-43.6415, 12.975) -> (-44.9549, 10.7)
  line L451 (-48.2747, 5.75) -> (-45.6478, 5.75)
  line L452 (-45.6478, 5.75) -> (-44.3343, 8.025)
  line L453 (-44.3343, 8.025) -> (-45.6478, 10.3)
  line L454 (-45.6478, 10.3) -> (-48.2747, 10.3)
  line L455 (-49.5882, 8.025) -> (-48.2747, 5.75)
  line L456 (-48.2747, 10.3) -> (-49.5882, 8.025)
  line L457 (-44.9549, 5.35) -> (-43.6415, 3.075)
  line L458 (-43.6415, 3.075) -> (-41.0145, 3.075)
  line L459 (-41.0145, 3.075) -> (-39.7011, 5.35)
  line L460 (-39.7011, 5.35) -> (-41.0145, 7.625)
  line L461 (-43.6415, 7.625) -> (-44.9549, 5.35)
  line L462 (-41.0145, 7.625) -> (-43.6415, 7.625)
  line L463 (-48.2747, 0.4) -> (-45.6478, 0.4)
  line L464 (-45.6478, 0.4) -> (-44.3343, 2.675)
  line L465 (-44.3343, 2.675) -> (-45.6478, 4.95)
  line L466 (-45.6478, 4.95) -> (-48.2747, 4.95)
  line L467 (-49.5882, 2.675) -> (-48.2747, 0.4)
  line L468 (-48.2747, 4.95) -> (-49.5882, 2.675)
  line L469 (-43.6415, -2.275) -> (-41.0145, -2.275)
  line L470 (-41.0145, -2.275) -> (-39.7011, 0)
  line L471 (-39.7011, 0) -> (-41.0145, 2.275)
  line L472 (-41.0145, 2.275) -> (-43.6415, 2.275)
  line L473 (-44.9549, 0) -> (-43.6415, -2.275)
  line L474 (-43.6415, 2.275) -> (-44.9549, 0)
  line L475 (-48.2747, -0.4) -> (-49.5882, -2.675)
  line L476 (-49.5882, -2.675) -> (-48.2747, -4.95)
  line L477 (-48.2747, -4.95) -> (-45.6478, -4.95)
  line L478 (-45.6478, -4.95) -> (-44.3343, -2.675)
  line L479 (-45.6478, -0.4) -> (-48.2747, -0.4)
  line L480 (-44.3343, -2.675) -> (-45.6478, -0.4)
  line L481 (-43.6415, -7.625) -> (-41.0145, -7.625)
  line L482 (-41.0145, -7.625) -> (-39.7011, -5.35)
  line L483 (-39.7011, -5.35) -> (-41.0145, -3.075)
  line L484 (-41.0145, -3.075) -> (-43.6415, -3.075)
  line L485 (-44.9549, -5.35) -> (-43.6415, -7.625)
  line L486 (-43.6415, -3.075) -> (-44.9549, -5.35)
  line L487 (-48.2747, -5.75) -> (-49.5882, -8.025)
  line L488 (-49.5882, -8.025) -> (-48.2747, -10.3)
  line L489 (-48.2747, -10.3) -> (-45.6478, -10.3)
  line L490 (-45.6478, -10.3) -> (-44.3343, -8.025)
  line L491 (-45.6478, -5.75) -> (-48.2747, -5.75)
  line L492 (-44.3343, -8.025) -> (-45.6478, -5.75)
  line L493 (-43.6415, -12.975) -> (-41.0145, -12.975)
  line L494 (-41.0145, -12.975) -> (-39.7011, -10.7)
  line L495 (-39.7011, -10.7) -> (-41.0145, -8.425)
  line L496 (-41.0145, -8.425) -> (-43.6415, -8.425)
  line L497 (-44.9549, -10.7) -> (-43.6415, -12.975)
  line L498 (-43.6415, -8.425) -> (-44.9549, -10.7)
  line L499 (-52.9075, 8.425) -> (-50.2805, 8.425)
  line L500 (-50.2805, 8.425) -> (-48.9671, 10.7)
  line L501 (-48.9671, 10.7) -> (-50.2805, 12.975)
  line L502 (-50.2805, 12.975) -> (-52.9075, 12.975)
  line L503 (-54.2209, 10.7) -> (-52.9075, 8.425)
  line L504 (-52.9075, 12.975) -> (-54.2209, 10.7)
  line L505 (-57.5407, 5.75) -> (-54.9138, 5.75)
  line L506 (-54.9138, 5.75) -> (-53.6003, 8.025)
  line L507 (-53.6003, 8.025) -> (-54.9138, 10.3)
  line L508 (-54.9138, 10.3) -> (-57.5407, 10.3)
  line L509 (-58.8542, 8.025) -> (-57.5407, 5.75)
  line L510 (-57.5407, 10.3) -> (-58.8542, 8.025)
  line L511 (-54.2209, 5.35) -> (-52.9075, 3.075)
  line L512 (-52.9075, 3.075) -> (-50.2805, 3.075)
  line L513 (-50.2805, 3.075) -> (-48.9671, 5.35)
  line L514 (-48.9671, 5.35) -> (-50.2805, 7.625)
  line L515 (-52.9075, 7.625) -> (-54.2209, 5.35)
  line L516 (-50.2805, 7.625) -> (-52.9075, 7.625)
  line L517 (-57.5407, 0.4) -> (-54.9138, 0.4)
  line L518 (-54.9138, 0.4) -> (-53.6003, 2.675)
  line L519 (-53.6003, 2.675) -> (-54.9138, 4.95)
  line L520 (-54.9138, 4.95) -> (-57.5407, 4.95)
  line L521 (-58.8542, 2.675) -> (-57.5407, 0.4)
  line L522 (-57.5407, 4.95) -> (-58.8542, 2.675)
  line L523 (-52.9075, -2.275) -> (-50.2805, -2.275)
  line L524 (-50.2805, -2.275) -> (-48.9671, 0)
  line L525 (-48.9671, 0) -> (-50.2805, 2.275)
  line L526 (-50.2805, 2.275) -> (-52.9075, 2.275)
  line L527 (-54.2209, 0) -> (-52.9075, -2.275)
  line L528 (-52.9075, 2.275) -> (-54.2209, 0)
  line L529 (-57.5407, -0.4) -> (-58.8542, -2.675)
  line L530 (-58.8542, -2.675) -> (-57.5407, -4.95)
  line L531 (-57.5407, -4.95) -> (-54.9138, -4.95)
  line L532 (-54.9138, -4.95) -> (-53.6003, -2.675)
  line L533 (-54.9138, -0.4) -> (-57.5407, -0.4)
  line L534 (-53.6003, -2.675) -> (-54.9138, -0.4)
  line L535 (-52.9075, -7.625) -> (-50.2805, -7.625)
  line L536 (-50.2805, -7.625) -> (-48.9671, -5.35)
  line L537 (-48.9671, -5.35) -> (-50.2805, -3.075)
  line L538 (-50.2805, -3.075) -> (-52.9075, -3.075)
  line L539 (-54.2209, -5.35) -> (-52.9075, -7.625)
  line L540 (-52.9075, -3.075) -> (-54.2209, -5.35)
  line L541 (-57.5407, -5.75) -> (-58.8542, -8.025)
  line L542 (-58.8542, -8.025) -> (-57.5407, -10.3)
  line L543 (-57.5407, -10.3) -> (-54.9138, -10.3)
  line L544 (-54.9138, -10.3) -> (-53.6003, -8.025)
  line L545 (-54.9138, -5.75) -> (-57.5407, -5.75)
  line L546 (-53.6003, -8.025) -> (-54.9138, -5.75)
  line L547 (-52.9075, -12.975) -> (-50.2805, -12.975)
  line L548 (-50.2805, -12.975) -> (-48.9671, -10.7)
  line L549 (-48.9671, -10.7) -> (-50.2805, -8.425)
  line L550 (-50.2805, -8.425) -> (-52.9075, -8.425)
  line L551 (-54.2209, -10.7) -> (-52.9075, -12.975)
  line L552 (-52.9075, -8.425) -> (-54.2209, -10.7)
  line L553 (-62.1735, 8.425) -> (-59.5465, 8.425)
  line L554 (-59.5465, 8.425) -> (-58.2331, 10.7)
  line L555 (-58.2331, 10.7) -> (-59.5465, 12.975)
  line L556 (-59.5465, 12.975) -> (-62.1735, 12.975)
  line L557 (-63.4869, 10.7) -> (-62.1735, 8.425)
  line L558 (-62.1735, 12.975) -> (-63.4869, 10.7)
  line L559 (-66.8067, 5.75) -> (-64.1798, 5.75)
  line L560 (-64.1798, 5.75) -> (-62.8663, 8.025)
  line L561 (-62.8663, 8.025) -> (-64.1798, 10.3)
  line L562 (-64.1798, 10.3) -> (-66.8067, 10.3)
  line L563 (-68.1202, 8.025) -> (-66.8067, 5.75)
  line L564 (-66.8067, 10.3) -> (-68.1202, 8.025)
  line L565 (-63.4869, 5.35) -> (-62.1735, 3.075)
  line L566 (-62.1735, 3.075) -> (-59.5465, 3.075)
  line L567 (-59.5465, 3.075) -> (-58.2331, 5.35)
  line L568 (-58.2331, 5.35) -> (-59.5465, 7.625)
  line L569 (-62.1735, 7.625) -> (-63.4869, 5.35)
  line L570 (-59.5465, 7.625) -> (-62.1735, 7.625)
  line L571 (-66.8067, 0.4) -> (-64.1798, 0.4)
  line L572 (-64.1798, 0.4) -> (-62.8663, 2.675)
  line L573 (-62.8663, 2.675) -> (-64.1798, 4.95)
  line L574 (-64.1798, 4.95) -> (-66.8067, 4.95)
  line L575 (-68.1202, 2.675) -> (-66.8067, 0.4)
  line L576 (-66.8067, 4.95) -> (-68.1202, 2.675)
  line L577 (-62.1735, -2.275) -> (-59.5465, -2.275)
  line L578 (-59.5465, -2.275) -> (-58.2331, 0)
  line L579 (-58.2331, 0) -> (-59.5465, 2.275)
  line L580 (-59.5465, 2.275) -> (-62.1735, 2.275)
  line L581 (-63.4869, 0) -> (-62.1735, -2.275)
  line L582 (-62.1735, 2.275) -> (-63.4869, 0)
  line L583 (-66.8067, -0.4) -> (-68.1202, -2.675)
  line L584 (-68.1202, -2.675) -> (-66.8067, -4.95)
  line L585 (-66.8067, -4.95) -> (-64.1798, -4.95)
  line L586 (-64.1798, -4.95) -> (-62.8663, -2.675)
  line L587 (-64.1798, -0.4) -> (-66.8067, -0.4)
  line L588 (-62.8663, -2.675) -> (-64.1798, -0.4)
  line L589 (-62.1735, -7.625) -> (-59.5465, -7.625)
  line L590 (-59.5465, -7.625) -> (-58.2331, -5.35)
  line L591 (-58.2331, -5.35) -> (-59.5465, -3.075)
  line L592 (-59.5465, -3.075) -> (-62.1735, -3.075)
  line L593 (-63.4869, -5.35) -> (-62.1735, -7.625)
  line L594 (-62.1735, -3.075) -> (-63.4869, -5.35)
  line L595 (-66.8067, -5.75) -> (-68.1202, -8.025)
  line L596 (-68.1202, -8.025) -> (-66.8067, -10.3)
  line L597 (-66.8067, -10.3) -> (-64.1798, -10.3)
  line L598 (-64.1798, -10.3) -> (-62.8663, -8.025)
  line L599 (-64.1798, -5.75) -> (-66.8067, -5.75)
  line L600 (-62.8663, -8.025) -> (-64.1798, -5.75)
  line L601 (-62.1735, -12.975) -> (-59.5465, -12.975)
  line L602 (-59.5465, -12.975) -> (-58.2331, -10.7)
  line L603 (-58.2331, -10.7) -> (-59.5465, -8.425)
  line L604 (-59.5465, -8.425) -> (-62.1735, -8.425)
  line L605 (-63.4869, -10.7) -> (-62.1735, -12.975)
  line L606 (-62.1735, -8.425) -> (-63.4869, -10.7)
  line L607 (-71.4395, 8.425) -> (-68.8125, 8.425)
  line L608 (-68.8125, 8.425) -> (-67.4991, 10.7)
  line L609 (-67.4991, 10.7) -> (-68.8125, 12.975)
  line L610 (-68.8125, 12.975) -> (-71.4395, 12.975)
  line L611 (-72.7529, 10.7) -> (-71.4395, 8.425)
  line L612 (-71.4395, 12.975) -> (-72.7529, 10.7)
  line L613 (-76.0727, 5.75) -> (-73.4458, 5.75)
  line L614 (-73.4458, 5.75) -> (-72.1323, 8.025)
  line L615 (-72.1323, 8.025) -> (-73.4458, 10.3)
  line L616 (-73.4458, 10.3) -> (-76.0727, 10.3)
  line L617 (-77.3862, 8.025) -> (-76.0727, 5.75)
  line L618 (-76.0727, 10.3) -> (-77.3862, 8.025)
  line L619 (-72.7529, 5.35) -> (-71.4395, 3.075)
  line L620 (-71.4395, 3.075) -> (-68.8125, 3.075)
  line L621 (-68.8125, 3.075) -> (-67.4991, 5.35)
  line L622 (-67.4991, 5.35) -> (-68.8125, 7.625)
  line L623 (-71.4395, 7.625) -> (-72.7529, 5.35)
  line L624 (-68.8125, 7.625) -> (-71.4395, 7.625)
  line L625 (-76.0727, 0.4) -> (-73.4458, 0.4)
  line L626 (-73.4458, 0.4) -> (-72.1323, 2.675)
  line L627 (-72.1323, 2.675) -> (-73.4458, 4.95)
  line L628 (-73.4458, 4.95) -> (-76.0727, 4.95)
  line L629 (-77.3862, 2.675) -> (-76.0727, 0.4)
  line L630 (-76.0727, 4.95) -> (-77.3862, 2.675)
  line L631 (-71.4395, -2.275) -> (-68.8125, -2.275)
  line L632 (-68.8125, -2.275) -> (-67.4991, 0)
  line L633 (-67.4991, 0) -> (-68.8125, 2.275)
  line L634 (-68.8125, 2.275) -> (-71.4395, 2.275)
  line L635 (-72.7529, 0) -> (-71.4395, -2.275)
  line L636 (-71.4395, 2.275) -> (-72.7529, 0)
  line L637 (-76.0727, -0.4) -> (-77.3862, -2.675)
  line L638 (-77.3862, -2.675) -> (-76.0727, -4.95)
  line L639 (-76.0727, -4.95) -> (-73.4458, -4.95)
  line L640 (-73.4458, -4.95) -> (-72.1323, -2.675)
  line L641 (-73.4458, -0.4) -> (-76.0727, -0.4)
  line L642 (-72.1323, -2.675) -> (-73.4458, -0.4)
  line L643 (-71.4395, -7.625) -> (-68.8125, -7.625)
  line L644 (-68.8125, -7.625) -> (-67.4991, -5.35)
  line L645 (-67.4991, -5.35) -> (-68.8125, -3.075)
  line L646 (-68.8125, -3.075) -> (-71.4395, -3.075)
  line L647 (-72.7529, -5.35) -> (-71.4395, -7.625)
  line L648 (-71.4395, -3.075) -> (-72.7529, -5.35)
  line L649 (-76.0727, -5.75) -> (-77.3862, -8.025)
  line L650 (-77.3862, -8.025) -> (-76.0727, -10.3)
  line L651 (-76.0727, -10.3) -> (-73.4458, -10.3)
  line L652 (-73.4458, -10.3) -> (-72.1323, -8.025)
  line L653 (-73.4458, -5.75) -> (-76.0727, -5.75)
  line L654 (-72.1323, -8.025) -> (-73.4458, -5.75)
  line L655 (-71.4395, -12.975) -> (-68.8125, -12.975)
  line L656 (-68.8125, -12.975) -> (-67.4991, -10.7)
  line L657 (-67.4991, -10.7) -> (-68.8125, -8.425)
  line L658 (-68.8125, -8.425) -> (-71.4395, -8.425)
  line L659 (-72.7529, -10.7) -> (-71.4395, -12.975)
  line L660 (-71.4395, -8.425) -> (-72.7529, -10.7)
  line L661 (-74.7592, -10.3) -> (-74.7592, -10.7)
  line L662 (-74.7592, -10.3) -> (-74.7592, 10.7)
  point P0 (-81, 0)
  point P1 (31.8, 0)
  point P2 (31.8, -5.35)
  point P3 (31.8, -10.7)
  point P4 (31.8, 5.35)
  point P5 (31.8, 10.7)
  point P6 (27.1668, -8.025)
  point P7 (27.1668, -2.675)
  point P8 (27.1668, 2.675)
  point P9 (27.1668, 8.025)
  dimension "d3" = 6
  dimension "d4" = 2
  dimension "d5" = 2
  dimension "d6" = 2
  dimension "d7" = 2.275
  dimension "d8" = 2.275
  dimension "d9" = 2.275
  dimension "d10" = 0.8
  dimension "d11" = 0.9
  dimension "d12" = 2.275
  dimension "d13" = 2.275
  dimension "d14" = 0.8
  dimension "d15" = 0.8
  dimension "d20" = 0.4
  dimension "d21" = 0.4
  dimension "d25" = 4.6332
  dimension "d33" = 0
  dimension "d34" = 9.266
  constraint horizontal L0
  constraint vertical L1
  constraint horizontal L2
  constraint vertical L3
  constraint midpoint L0 L5.start
  constraint midpoint L2 L5.end
  constraint midpoint L3 P1
  constraint perpendicular L3 L14
  constraint midpoint L1 L15.end
  constraint perpendicular L1 L15
  constraint coincident P1 L15
  constraint coincident L3 P1
  constraint coincident L3 P2
  constraint parallel L0 L23
  constraint coincident L3 P3
  constraint coincident L0 P3
  constraint coincident L3 P4
  constraint coincident L2 P5
  constraint coincident L3 P5
  constraint coincident L0 L64.start
  constraint coincident L2 L64.end
  constraint perpendicular L2 L64
  constraint parallel L0 L41
  constraint parallel L0 L50
  constraint coincident P6 L64
  constraint coincident P7 L64
  constraint coincident P8 L64
  constraint coincident P9 L64
  constraint midpoint L651 L661.start
  constraint coincident L0 L661.end
  constraint perpendicular L0 L661
  constraint coincident L2 L662.end
  constraint perpendicular L2 L662
  measures "d3" distance of L1 P0
  measures "d4" distance of L3 L4
  measures "d5" distance of L2 L6
  measures "d6" distance of L0 L7
  measures "d7" distance of P1 L13
  measures "d8" distance of P2 L21
  measures "d9" distance of P3 L27
  measures "d10" distance of L18 L26
  measures "d12" distance of P4 L33
  measures "d13" distance of P5 L39
  measures "d14" distance of L32 L36
  measures "d15" distance of L12 L29
  measures "d20" distance of L0 L41
  measures "d21" distance of L15 L50
  measures "d25" distance of L3 L64
extrude "Extrude15" cut sketch "Sketch10" against normal through all contours L0 L3 L26 L27 | L0 L117 L118 L120 | L3 L16 L17 L18 L21 | L0 L171 L172 L174 | L3 L8 L9 L14 | L3 L12 L13 L14 | L0 L225 L226 L228 | L3 L28 L29 L32 L33 | L0 L279 L280 L282 | L2 L3 L35 L36 | L0 L333 L334 L336 | L0 L387 L388 L390 | L2 L67 L68 L71 | L0 L441 L442 L444 | L2 L121 L122 L125 | L0 L495 L496 L498 | L2 L175 L176 L179 | L0 L549 L550 L552 | L2 L229 L230 L233 | L0 L603 L604 L606 | L2 L283 L284 L287 | L0 L657 L658 L660 | L2 L337 L338 L341 | L2 L391 L392 L395 | L651 L652 L653 L654 L662 | L2 L445 L446 L449 | L639 L640 L641 L642 L662 | L2 L499 L500 L503 | L625 L626 L627 L628 L662 | L2 L553 L554 L557 | L613 L614 L615 L616 L662 | L2 L607 L608 L611 | L40 L41 L42 L43 L44 L45 | L46 L47 L48 L49 L50 L51 | L52 L53 L54 L55 L56 L57 | L58 L59 L60 L61 L62 L63 | L65 L163 L164 L165 L166 L167 L168 | L66 L217 L218 L219 L220 L221 L222 | L73 L74 L75 L76 L77 L78 | L79 L80 L81 L82 L83 L84 | L85 L86 L87 L88 L89 L90 | L91 L92 L93 L94 L95 L96 | L97 L98 L99 L100 L101 L102 | L103 L104 L105 L106 L107 L108 | L109 L110 L111 L112 L113 L114 | L127 L128 L129 L130 L131 L132 | L133 L134 L135 L136 L137 L138 | L139 L140 L141 L142 L143 L144 | L145 L146 L147 L148 L149 L150 | L151 L152 L153 L154 L155 L156 | L157 L158 L159 L160 L161 L162 | L181 L182 L183 L184 L185 L186 | L187 L188 L189 L190 L191 L192 | L193 L194 L195 L196 L197 L198 | L199 L200 L201 L202 L203 L204 | L205 L206 L207 L208 L209 L210 | L211 L212 L213 L214 L215 L216 | L235 L236 L237 L238 L239 L240 | L241 L242 L243 L244 L245 L246 | L247 L248 L249 L250 L251 L252 | L253 L254 L255 L256 L257 L258 | L259 L260 L261 L262 L263 L264 | L265 L266 L267 L268 L269 L270 | L271 L272 L273 L274 L275 L276 | L289 L290 L291 L292 L293 L294 | L295 L296 L297 L298 L299 L300 | L301 L302 L303 L304 L305 L306 | L307 L308 L309 L310 L311 L312 | L313 L314 L315 L316 L317 L318 | L319 L320 L321 L322 L323 L324 | L325 L326 L327 L328 L329 L330 | L343 L344 L345 L346 L347 L348 | L349 L350 L351 L352 L353 L354 | L355 L356 L357 L358 L359 L360 | L361 L362 L363 L364 L365 L366 | L367 L368 L369 L370 L371 L372 | L373 L374 L375 L376 L377 L378 | L379 L380 L381 L382 L383 L384 | L397 L398 L399 L400 L401 L402 | L403 L404 L405 L406 L407 L408 | L409 L410 L411 L412 L413 L414 | L415 L416 L417 L418 L419 L420 | L421 L422 L423 L424 L425 L426 | L427 L428 L429 L430 L431 L432 | L433 L434 L435 L436 L437 L438 | L451 L452 L453 L454 L455 L456 | L457 L458 L459 L460 L461 L462 | L463 L464 L465 L466 L467 L468 | L469 L470 L471 L472 L473 L474 | L475 L476 L477 L478 L479 L480 | L481 L482 L483 L484 L485 L486 | L487 L488 L489 L490 L491 L492 | L505 L506 L507 L508 L509 L510 | L511 L512 L513 L514 L515 L516 | L517 L518 L519 L520 L521 L522 | L523 L524 L525 L526 L527 L528 | L529 L530 L531 L532 L533 L534 | L535 L536 L537 L538 L539 L540 | L541 L542 L543 L544 L545 L546 | L559 L560 L561 L562 L563 L564 | L565 L566 L567 L568 L569 L570 | L571 L572 L573 L574 L575 L576 | L577 L578 L579 L580 L581 L582 | L583 L584 L585 L586 L587 L588 | L589 L590 L591 L592 L593 L594 | L595 L596 L597 L598 L599 L600 | L619 L620 L621 L622 L623 L624 | L631 L632 L633 L634 L635 L636 | L643 L644 L645 L646 L647 L648
equation "d22_3_1 = d21_3_1 / 2"
equation "d24_3_1 = d23_3_1 / 2"
equation "d26_3_1 = d25_3_1"
equation "d27_3_1 = d25_3_1"
equation "d28_3_1 = d25_3_1"
equation "d33_3_1 = d32_3_1"
equation "d6 = d5"
equation "d8 = d7"
equation "d9 = d7"
equation "d12 = d7"
equation "d13 = d7"
